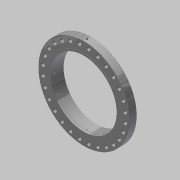
# Autodesk Inventor part: A1-19037-100-04 28in CL300 RF flange - custom
Saved by Autodesk Inventor 2017.3 (Build 213257000, 257)
## iProperties
Created: 2011-05-31
Part Number: A1-19037-100-04 28in CL300 RF flange - custom
Document SubType Name: Modeling
Designer: Graeme_Van_Dongen
Density: 7.85 g/cm^3
Description: 28" CLASS 300 B16.47 Ser.A RFSO FLANGE, A105N, Ø28 7/8" BORE
Material: Steel
Mass: 277806 g
Surface Area: 17766.4 cm^2
Volume: 35389.3 cm^3
Appearance: Steel
Project: A1-19037--CNUL Albian CST laterals
Constructed By: Graeme_Van_Dongen
Project Name: CST laterals
Author: Graeme_Van_Dongen
Autodesk Inventor part; units mm, degrees
ref_plane "YZ Plane" through (0, 0, 0) normal (1, 0, 0) x (0, 1, 0)
ref_plane "XY Plane" through (0, 0, 0) normal (0, 0, 1) x (1, 0, 0)
sketch "Sketch1" plane through (0, 0, 0) normal (0, 0, 1) x (1, 0, 0)
  circle A0 centre (0, 0) radius 517.525
  circle A1 centre (0, 0) radius 371.475
  dimension "d0" = 1035.05
  dimension "d1" = 742.95
  constraints: 2 centre point, 2 coincident
  measures "d0" diameter of A0
  measures "d1" diameter of A1
extrude "Extrusion1" add sketch "Sketch1" along normal blind 84.1375
sketch "Sketch2" plane through (0, 0, 84.1375) normal (0, 0, 1) x (1, 0, 0)
  circle A0 centre (0, 0) radius 371.475 projected
  circle A1 centre (0, 0) radius 517.525 projected
  circle A2 centre (0, 0) radius 400.05
  dimension "d4" = 800.1
  constraints: 1 centre point, 1 coincident
  measures "d4" diameter of A2
extrude "Extrusion2" add sketch "Sketch2" along normal blind 1.5875 contours A2
sketch "Sketch3" plane through (0, 0, 0) normal (0, 0, -1) x (-1, 0, 0)
  circle A0 centre (0, 0) radius 371.475 projected
  circle A1 centre (0, 0) radius 517.525 projected
  circle A2 centre (0, 0) radius 415.925
  dimension "d7" = 831.85
  constraints: 1 centre point, 1 coincident
  measures "d7" diameter of A2
extrude "Extrusion3" add sketch "Sketch3" along normal blind 57.15 contours A2
sketch "Sketch4" plane through (0, 0, 85.725) normal (0, 0, 1) x (1, 0, 0)
  line L0 (0, 0) -> (52.6121, 466.9454) construction
  line L1 (0, -724.535) -> (0, 724.535) construction
  dimension "d13" = 469.9
  dimension "d99" = 6.429
  constraints: 2 end point
  measures "d13" distance of L0.start L0.end
  measures "d99" angle of L0 L1
hole "Hole1" at (52.6121, 466.9454, 85.725) direction (0, 0, -1) diameter 44.45 end through all
chamfer "Chamfer3" distance 0.7937 angle 45 2 edges at (52.6121, 489.1704, 0) (52.6121, 489.1704, 84.1375)
pattern_circular "Circular Pattern1" count 28 over 360 about axis through (0, 0, -10) along (0, 0, -1) of "Hole1", "Chamfer3"
chamfer "Chamfer2" distance 1.5875 angle 45 2 edges at (-517.525, 0, 0) (-517.525, 0, 84.1375)
fillet "Fillet2" radius 11.1125 1 edges at (415.925, 0, 0)
chamfer "Chamfer4" distance 1.5875 angle 45 1 edges at (415.925, 0, -57.15)
sketch "Sketch6" plane through (0, 0, 0) normal (1, 0, 0) x (0, 1, 0)
  line L0 (415.925, -11.1125) -> (415.925, -55.5625) construction
  line L1 (414.3375, -57.15) -> (-414.3375, -57.15) construction
  line L2 (406.4, -37.4006) -> (388.9375, -50.8)
  line L3 (385.7625, -57.15) -> (415.925, -57.15)
  line L4 (0, -85.725) -> (0, 114.3) projected
  line L5 (385.7625, -57.15) -> (385.7625, -50.8)
  line L6 (371.475, -57.15) -> (371.475, 85.725) construction
  line L7 (385.7625, -50.8) -> (388.9375, -50.8)
  line L8 (371.475, 85.725) -> (374.65, 85.725)
  line L9 (374.65, 85.725) -> (374.65, 60.325)
  line L10 (374.65, 60.325) -> (371.475, 60.325)
  line L11 (371.475, 60.325) -> (371.475, 85.725)
  line L12 (406.4, -37.4006) -> (406.4, -31.75)
  line L13 (415.925, -19.4533) -> (415.925, -57.15)
  arc A0 (415.925, -19.4533) -> (406.4, -31.75) centre (419.1, -31.75) ccw
  point P0 (0, 0)
  dimension "d45" = 37.5
  dimension "d59" = 6.35
  dimension "d69" = 17.4625
  dimension "d70" = 3.175
  dimension "d71" = 25.4
  dimension "d72" = 374.65
  dimension "d96" = 406.4
  dimension "d97" = 12.7
  dimension "d98" = 25.4
  constraints: 21 end point, 3 collinear, 3 parallel, 2 horizontal, 2 point on circle, 2 point on line, 1 centre point, 1 perpendicular, 1 tangent, 1 vertical
  measures "d45" angle of L3 L2
  measures "d59" distance of L3.start L5.end
  measures "d69" horizontal distance of L2.start L2.end
  measures "d70" distance of L5.end L2.end
  measures "d71" distance from line of L6.end L10
  measures "d72" distance from line of point (0, 0) L9
  measures "d96" distance between parallel lines of L4 L12
  measures "d97" radius of A0
  measures "d98" distance from line of A0.centre L3
revolve "Revolution1" cut sketch "Sketch6" angle 360 about axis through (0, 0, -10) along (0, 0, 1)
fillet "Fillet5" radius 0.7937 1 edges at (0, -374.65, 60.325)
chamfer "Chamfer7" distance 0.7937 angle 45 1 edges at (-371.475, 0, 60.325)
ref_plane "Work Plane1" through (0, 517.525, 0) normal (0, 1, 0) x (-1, 0, 0)
sketch "Sketch11" plane through (0, 517.525, 0) normal (0, 1, 0) x (-1, 0, 0)
  line L0 (-373.8563, 60.325) -> (373.8563, 60.325) construction
  line L1 (372.2688, 60.325) -> (-372.2688, 60.325) construction
  point P0 (0, 0)
  point P1 (0, 47.625)
  dimension "d101" = 12.7
  constraints: 1 vertical alignment
  measures "d101" distance from line of L0 point (0, 47.625)
hole "Hole4" at (0, 517.525, 47.625) direction (0, -1, 0) diameter 17.4752 depth 27.94 tip angle 118 thread size "1/2" designation "1/2 - 14 NPT" standard "NPT"
hole "Hole5" at (0, 517.525, 47.625) direction (0, -1, 0) diameter 10.5918 depth 44.45 tip angle 118 thread size "1/2-13 UNC" class "2B" standard "ANSI Unified Screw Threads"
hole "Hole6" at (0, 517.525, 47.625) direction (0, -1, 0) diameter 10.3188 depth 152.4 tip angle 118
pattern_circular "Circular Pattern3" count 4 over 360 about axis through (0, 0, -10) along (0, 0, 1) of "Hole4", "Hole5", "Hole6"
equation "\"d0\" = OD"
equation "\"d1\" = Bore"
equation "\"d2\" = Thickness"
equation "\"d4\" = RFDia"
equation "\"d5\" = RFDepth"
equation "\"d7\" = NeckDia"
equation "\"d8\" = NeckLength"
equation "\"d13\" = 0.5 * BCD"
equation "\"d15\" = HoleDia"
equation "\"d30\" = HoleChamfer"
equation "\"d25\" = RimChamfer"
equation "\"d29\" = NeckFillet"
equation "\"d33\" = NeckChamfer"
equation "\"d72\" = 0.5 * Bore + Lockstep"
equation "\"d96\" = 0.5 * Casing"
equation "\"OD\" = 1035.05"
equation "\"Bore\" = 742.95"
equation "\"Thickness\" = 84.1375"
equation "\"RFDia\" = 800.1"
equation "\"RFDepth\" = 1.5875"
equation "\"HoleDia\" = 44.45"
equation "\"BCD\" = 939.8"
equation "\"NeckDia\" = 831.85"
equation "\"HoleChamfer\" = 0.79375"
equation "\"RimChamfer\" = 1.5875"
equation "\"NeckChamfer\" = 1.5875"
equation "\"NeckFillet\" = 11.1125"
equation "\"Lock\" = 25.4"
equation "\"Lockstep\" = 3.175"
equation "\"Size\" = 711.2"
equation "\"Wall\" = 19.05"
equation "\"NeckLength\" = 57.15"
equation "\"Casing\" = 812.8"
body "Solid1"
